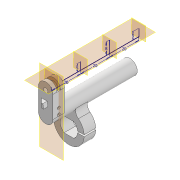
# Autodesk Inventor part: base_hand
Saved by Autodesk Inventor 2020.2 (Build 242310000, 310)
## iProperties
Created: 2020-04-08
Part Number: base_hand
Material: Generic
Document SubType Name: Modeling
Designer: Bardo91
Density: 1 g/cm^3
Appearance: Default
Author: Bardo91
Autodesk Inventor part; units mm, degrees
ref_plane "YZ Plane" through (0, 0, 0) normal (1, 0, 0) x (0, 1, 0)
sketch "Sketch1" plane through (0, 0, 0) normal (1, 0, 0) x (0, 1, 0)
  line L0 (0, 0) -> (0, -20)
  line L1 (0, -20) -> (0, -40)
  line L2 (0, -40) -> (0, -60)
  line L3 (0, -20) -> (5, -20)
  line L4 (0, -40) -> (8, -40)
  line L5 (0, -60) -> (5, -60)
  dimension "d0" = 20
  dimension "d1" = 20
  dimension "d2" = 20
  dimension "d4" = 5
  dimension "d5" = 8
  dimension "d6" = 5
  constraints: 12 end point, 2 horizontal, 2 point on line, 1 perpendicular, 1 vertical
  measures "d0" distance of L0.start L0.end
  measures "d1" distance of L0.end L1.end
  measures "d2" distance of L1.end L2.end
  measures "d4" distance of L0.end L3.end
  measures "d5" distance of L1.end L4.end
  measures "d6" distance of L2.end L5.end
ref_plane "Work Plane1" through (0, 5, -20) normal (0, 0, 1) x (1, 0, 0)
ref_plane "Work Plane3" through (0, 5, -60) normal (0, 0, 1) x (1, 0, 0)
ref_plane "Work Plane2" through (0, 8, -40) normal (0, 0, 1) x (1, 0, 0)
ref_plane "Work Plane4" through (0, 0, 0) normal (0, 0, 1) x (1, 0, 0)
sketch "Sketch2" plane through (0, 0, 0) normal (0, 0, 1) x (1, 0, 0)
  circle A0 centre (0, 0) radius 1.5
  circle A1 centre (0, 0) radius 5
  line L0 (0, 0) -> (0, -15)
  circle A2 centre (0, -15) radius 5
  line L1 (5, -15) -> (5, 0)
  line L2 (-5, -15) -> (-5, 0)
  dimension "d7" = 3
  dimension "d8" = 10
  dimension "d80" = 15
  dimension "d81" = 10
  constraints: 6 end point, 4 point on circle, 3 centre point, 3 coincident, 2 tangent, 2 vertical, 1 parallel
  measures "d7" diameter of A0
  measures "d8" diameter of A1
  measures "d80" distance of L0.start L0.end
  measures "d81" diameter of A2
extrude "pinky_joint" add sketch "Sketch2" along normal mid plane 8
sketch "Sketch18" plane through (0, 0, 4) normal (0, 0, 1) x (1, 0, 0)
  line L0 (0, 0) -> (0, -6)
  line L1 (0, -6) -> (0, -9)
  line L2 (0, 0) -> (1.058, -6)
  line L3 (0, 0) -> (6.0926, 0) construction
  line L4 (1.058, -6) -> (0, -6)
  line L5 (1.058, -6) -> (1.5869, -9)
  line L6 (1.5869, -9) -> (0, -9)
  dimension "d82" = 6
  dimension "d83" = 3
  dimension "d84" = 80
  constraints: 14 end point, 2 horizontal, 2 point on line, 1 equal length, 1 parallel, 1 vertical
  measures "d82" distance of L0.start L0.end
  measures "d83" distance of L0.end L1.end
  measures "d84" angle of L2 L3
extrude "lock" add sketch "Sketch18" along normal blind 3 contours L4 L5 L6 L1
ref_plane "Work Plane5" through (0, 0, 0) normal (0, 0, 1) x (1, 0, 0)
mirror "Mirror1" about plane through (0, 0, 0) normal (0, 0, 1) of "lock"
chamfer "Chamfer1" distance 3 angle 45 2 edges at (0, -7.5, 4) (0, -7.5, -4)
ref_plane "Work Plane6" through (0, 5, 0) normal (0, 1, 0) x (-1, 0, 0)
sketch "Sketch19" plane through (0, 5, 0) normal (0, 1, 0) x (-1, 0, 0)
  line L0 (0, 0) -> (-3, 0)
  circle A0 centre (-3, 0) radius 1.25
  dimension "d90" = 3
  dimension "thread_hole" = 2.5
  constraints: 2 end point, 1 centre point, 1 coincident, 1 horizontal
  measures "d90" distance of L0.start L0.end
  measures "thread_hole" diameter of A0
extrude "thread_hole" cut sketch "Sketch19" against normal through all
sketch "Sketch20" plane through (0, 0, 0) normal (0, 1, 0) x (-1, 0, 0)
  line L0 (0, 0) -> (-3, 0)
  circle A0 centre (-3, 0) radius 1.25
  line L1 (-3, -1.25) -> (-5, -1.25)
  line L2 (-5, -4) -> (-5, 4) projected
  line L3 (-3, 1.25) -> (-5, 1.25)
  line L4 (0, 0) -> (0, 2.405)
  dimension "d94" = 3
  dimension "d95" = 2.5
  constraints: 8 end point, 2 horizontal, 2 point on circle, 2 point on line, 1 centre point, 1 coincident, 1 parallel, 1 vertical
  measures "d94" distance of L0.start L0.end
  measures "d95" diameter of A0
revolve "Revolution2" cut sketch "Sketch20" angle 180 about axis through (0, 0, 0) along (0, 0, 1)
sketch "Sketch22" plane through (5, -15, 4) normal (1, 0, 0) x (0, 0, -1)
  line L0 (8, 0) -> (0, 0) projected
  line L1 (4, 0) -> (4, 1)
  circle A0 centre (4, 1) radius 1
  line L2 (4, 1) -> (4, 5)
  circle A1 centre (4, 5) radius 1
  point P0 (4, 15)
  dimension "d100" = 1
  dimension "d101" = 2
  dimension "d104" = 4
  dimension "d105" = 2
  constraints: 4 end point, 2 centre point, 2 coincident, 2 vertical, 1 midpoint
  measures "d100" distance of L1.start L1.end
  measures "d101" diameter of A0
  measures "d104" distance of L2.start L2.end
  measures "d105" diameter of A1
extrude "flector_holder" cut sketch "Sketch22" against normal up to surface round surface about axis through (3, 5, 0) along (0, -1, 0) radius 1.25 far side no
sketch "Sketch23" plane through (0, 0, -4) normal (0, 0, -1) x (-1, 0, 0)
  arc A0 (-5, -15) -> (5, -15) centre (0, -15) ccw projected
  circle A1 centre (0, -15) radius 5
  point P0 (0, 0)
  constraints: 1 coincident, 3 other
extrude "Extrusion15" add sketch "Sketch23" along normal blind 50
sketch "Sketch7" plane through (0, 5, -20) normal (0, 0, 1) x (1, 0, 0)
  arc A0 (5, -5) -> (-5, -5) centre (0, -5) ccw projected
  line L0 (0, -5) -> (0, -35)
  circle A1 centre (0, -35) radius 6
  circle A2 centre (0, -35) radius 10.5
  line L1 (0, -35) -> (0, -34.5)
  line L2 (0, -35) -> (0, -35.5)
  line L3 (0, -35.5) -> (10.4881, -35.5)
  line L4 (0, -34.5) -> (10.4766, -34.3)
  line L5 (0, -35) -> (0, -30)
  line L6 (0, -30) -> (3.3166, -30)
  line L7 (0, -30) -> (-3.3166, -30)
  line L8 (0, -35) -> (0, -40)
  line L9 (0, -40) -> (3.3166, -40)
  line L10 (0, -40) -> (-3.3166, -40)
  point P0 (5.9685, -34.3861)
  point P1 (5.9791, -35.5)
  dimension "d33" = 30
  dimension "d34" = 12
  dimension "d35" = 21
  dimension "d36" = 0.5
  dimension "d37" = 0.5
  dimension "d50" = 5
  dimension "d51" = 5
  constraints: 22 end point, 6 point on circle, 5 point on line, 3 perpendicular, 2 centre point, 2 coincident, 2 vertical
  measures "d33" distance of L0.start L0.end
  measures "d34" diameter of A1
  measures "d35" diameter of A2
  measures "d36" distance of L1.start L1.end
  measures "d37" distance of L1.start L2.end
  measures "d50" distance of L1.start L5.end
  measures "d51" distance of L1.start L8.end
extrude "pinky_motor" add sketch "Sketch7" along normal blind 8 contours L7 A1 L0 | L0 A1 L6 | A1 L3 A2 L0 | L0 A2 L4 A1 | L10 L9 A1
fillet "Fillet2" radius 5 2 edges at (1.8166, -19.6583, -16) (-1.8166, -19.6583, -16)
sketch "Sketch24" plane through (-5, 0, -1.25) normal (0, 1, 0) x (1, 0, 0)
  arc A0 (2, -2.5) -> (2, 0) centre (2, -1.25) ccw projected
  circle A1 centre (2, -1.25) radius 1.25
  point P0 (5, -1.25)
  constraints: 1 coincident, 3 other
extrude "Extrusion16" cut sketch "Sketch24" against normal through all
equation "\"d95\" = thread_hole"
body "Solid1"
